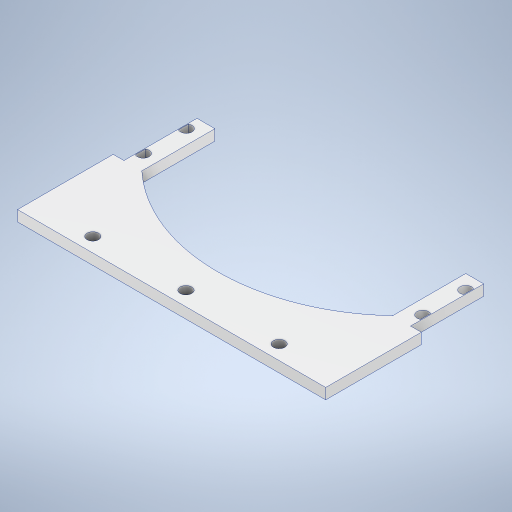
# Autodesk Inventor part: chest_cover_base
Saved by Autodesk Inventor 2024.1 (Build 281209000, 209)
## iProperties
Created: 2024-10-11
Part Number: chest_cover_base
Material: アルミニウム 6061
Document SubType Name: Sheet Metal
Designer: hibik
Density: 2.7 g/cm^3
Sheet Metal Rule: Default_mm
Appearance: アルミニウム - フラット
Author: hibik
Autodesk Inventor part; units mm, degrees
ref_plane "YZ Plane" through (0, 0, 0) normal (1, 0, 0) x (0, 1, 0)
ref_plane "XZ Plane" through (0, 0, 0) normal (0, 1, 0) x (-1, 0, 0)
ref_plane "XY Plane" through (0, 0, 0) normal (0, 0, 1) x (1, 0, 0)
sketch "スケッチ7" plane through (0, 1.5, 0) normal (0, 1, 0) x (1, 0, 0)
  line L0 (-20, 0) -> (-19.9, 0)
  line L1 (-19.9, 0) -> (-19.9, -10.2)
  line L2 (-19.9, -10.2) -> (-20, -10.2)
  line L3 (-20, -10.2) -> (-20, 0)
  line L4 (17.5, 0) -> (20, 0)
  line L5 (20, 0) -> (19.9, 0)
  line L6 (19.9, 0) -> (19.9, -10.2)
  line L7 (19.9, -10.2) -> (20, -10.2)
  line L8 (20, -10.2) -> (20, 0)
  line L9 (-20, -10.2) -> (-21.5, -10.2)
  line L10 (-20, 0) -> (-20, -1.3755)
  point P0 (0, 0)
  dimension "d21" = 0.1
  dimension "d22" = 0.1
  measures "d21" distance of L1.end L2.end
  measures "d22" distance of L7.end L6.end
sketch "スケッチ1" plane through (0, 0, 0) normal (0, 1, 0) x (-1, 0, 0)
  line L0 (21.5, 0) -> (-21.5, 0)
  line L1 (-21.5, 0) -> (-21.5, 25.1)
  line L2 (-21.5, 25.1) -> (21.5, 25.1)
  line L3 (21.5, 25.1) -> (21.5, 0)
  point P0 (0, 0)
  point P1 (0, 0)
  dimension "d0" = 25.1
  dimension "d1" = 43
  measures "d0" distance of L2.end L0.start
  measures "d1" distance of L0.start L0.end
extrude "プレート1" add sketch "スケッチ1" along normal blind 1.5
sketch "スケッチ3" plane through (0, 1.5, 0) normal (0, 1, 0) x (1, 0, 0)
  line L0 (21.5, 0) -> (-21.5, 0) projected
  line L1 (-20, 0) -> (-20, -17.1)
  line L2 (20, 0) -> (20, -17.1)
  line L3 (-21.5, -25.1) -> (-21.5, 0) projected
  line L4 (21.5, 0) -> (21.5, -25.1) projected
  line L5 (-20, -17.1) -> (20, -17.1)
  line L6 (-20, 0) -> (-17.5, 0)
  line L7 (-17.5, 0) -> (-17.5, -10.2)
  line L8 (-17.5, -10.2) -> (-20, -10.2)
  line L9 (-20, -10.2) -> (-20, 0)
  line L10 (20, 0) -> (17.5, 0)
  line L11 (17.5, 0) -> (17.5, -10.2)
  line L12 (17.5, -10.2) -> (20, -10.2)
  line L13 (20, -10.2) -> (20, 0)
  line L14 (-20, -10.2) -> (-21.5, -10.2)
  line L15 (20, -10.2) -> (21.5, -10.2)
  line L16 (21.5, -25.1) -> (-21.5, -25.1) projected
  arc A0 (-17.5, -10.2) -> (17.5, -10.2) centre (0, 8.542) ccw
  point P0 (0, 0)
  point P1 (20, -10.2)
  point P2 (17.5, 0)
  point P3 (-17.5, 0)
  dimension "d5" = 1.5
  dimension "d6" = 1.5
  dimension "d7" = 2.5
  dimension "d8" = 10.2
  dimension "d9" = 8
  constraints: 26 end point, 5 point on line, 4 horizontal, 4 parallel, 2 collinear, 2 perpendicular, 2 point on circle, 2 vertical, 1 centre point, 1 tangent
  measures "d5" distance between parallel lines of L3 L1
  measures "d6" distance between parallel lines of L4 L2
  measures "d7" distance of L7.end L8.end
  measures "d8" distance of L6.end L7.end
  measures "d9" distance between parallel lines of L5 L16
extrude "押し出し2" cut sketch "スケッチ3" against normal through all contours L4 L15 L2 L0 | L11 A0 L7 L0 | L1 L14 L3 L0
sketch "スケッチ4" plane through (-21.5, 0, 25.1) normal (-1, 0, 0) x (0, 0, 1)
  line L0 (-0.5569, 2.6) -> (-0.5569, 0)
  line L1 (0, 0) -> (-14.9, 0) projected
  line L2 (-14.9, 1.5) -> (-14.9, 0) projected
  line L3 (-14.9, 0) -> (0, 0) projected
  line L4 (0, 0) -> (0, 1.5) projected
  line L5 (0, 1.5) -> (-14.9, 1.5) projected
  point P0 (-25.1, 0)
  point P1 (0, 0)
  point P2 (-0.5569, 1.5)
  constraints: 2 end point, 1 point on line, 1 vertical, 1 other
extrude "押し出し3" cut sketch "スケッチ4" against normal through all contours L5 L4 L1 L0
sketch "スケッチ5" plane through (0, 1.5, 0) normal (0, 1, 0) x (1, 0, 0)
  circle A0 centre (0, -21.5431) radius 0.8 projected
  circle A1 centre (-13, -21.5431) radius 0.8 projected
  circle A2 centre (13, -21.5431) radius 0.8 projected
  line L0 (-21.5, -24.5431) -> (-21.5, -10.2) projected
  line L1 (-21.5, -23.5431) -> (21.5, -23.5431)
  line L2 (21.5, -24.5431) -> (-21.5, -24.5431) projected
  line L3 (21.5, -10.2) -> (21.5, -24.5431) projected
  point P0 (0, 0)
  dimension "d16" = 1
  constraints: 2 end point, 1 parallel, 1 point on line
  measures "d16" distance between parallel lines of L2 L1
extrude "切り取り1" cut sketch "スケッチ5" against normal blind 1.5
sketch "スケッチ6" plane through (0, 1.5, 0) normal (0, 1, 0) x (1, 0, 0)
  circle A0 centre (19.5, -2) radius 0.8 projected
  circle A1 centre (19.5, -8) radius 0.8 projected
  line L0 (0, -21.3988) -> (0, 0)
  circle A2 centre (-19.5, -2) radius 0.8
  circle A3 centre (-19.5, -8) radius 0.8
  line L1 (-20, 0) -> (-17.5, 0) projected
  line L2 (-20, 0) -> (-19.9, 0)
  line L3 (-19.9, 0) -> (-19.9, -10.2)
  line L4 (-19.9, -10.2) -> (-20, -10.2)
  line L5 (-20, -10.2) -> (-20, 0)
  line L6 (-20, -10.2) -> (-21.5, -10.2) projected
  line L7 (20, 0) -> (19.9, 0)
  line L8 (19.9, 0) -> (19.9, -10.2)
  line L9 (19.9, -10.2) -> (20, -10.2)
  line L10 (20, -10.2) -> (20, 0)
  line L11 (17.5, 0) -> (20, 0) projected
  line L12 (21.5, -10.2) -> (20, -10.2) projected
  line L13 (20, -10.2) -> (20, 0) projected
  dimension "d19" = 0.1
  dimension "d20" = 0.1
  constraints: 18 end point, 4 collinear, 4 parallel, 2 centre point, 2 horizontal, 2 perpendicular, 2 symmetric about line, 1 vertical, 2 other
  measures "d19" distance between parallel lines of L5 L3
  measures "d20" distance between parallel lines of L10 L8
extrude "切り取り2" cut sketch "スケッチ6" against normal blind 1.5 contours A0 L10 | L10 A0 L8 | L8 A0 | L10 A1 L8 | A1 L10 | L8 A1 | A2 L3 | L3 A2 L5 | L5 A2 | L3 A3 L5 | A3 L3 | L5 A3
sheet face with bend "面2" sketch "スケッチ7" thickness 1.5 toward (0, -1, 0) bend radius 1.5
bend "曲げ1"
equation "\"d6\" = d5"
equation "\"d14\" = Thickness"
equation "\"d17\" = Thickness"
equation "\"d2\" = Thickness"
equation "\"d23\" = BendRadius"
equation "\"d24\" = BendReliefWidth"
equation "\"d26\" = MinimumRemnant"
equation "\"d25\" = BendReliefDepth"
equation "\"d27\" = TransitionRadius"
equation "\"BendRadius\" = Thickness"
equation "\"BendReliefWidth\" = Thickness"
equation "\"BendReliefDepth\" = 0.5 * Thickness"
equation "\"CornerReliefSize\" = 4 * Thickness"
equation "\"MinimumRemnant\" = 2 * Thickness"
equation "\"TransitionRadius\" = BendRadius"
equation "\"JacobiRadiusSize\" = BendRadius"
equation "\"GapSize\" = Thickness"
equation "\"Thickness\" = 1.5"
